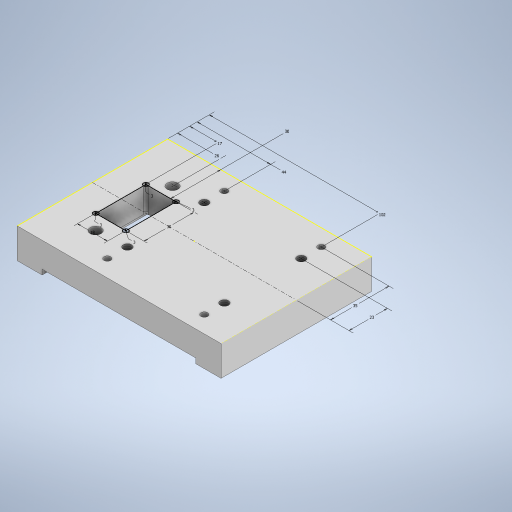
# Autodesk Inventor part: 05-15-2023 esercizi_iogna_serie
Saved by Autodesk Inventor 2023 (Build 270158000, 158)
## iProperties
Created: 2023-05-15
Part Number: 05-15-2023 esercizi_iogna_serie
Material: Generico
Document SubType Name: Modeling
Designer: Admin
Density: 1 g/cm^3
Appearance: Default
Author: Admin
Autodesk Inventor part; units mm, degrees
ref_plane "YZ Plane" through (0, 0, 0) normal (1, 0, 0) x (0, 1, 0)
ref_plane "XZ Plane" through (0, 0, 0) normal (0, 1, 0) x (-1, 0, 0)
ref_plane "XY Plane" through (0, 0, 0) normal (0, 0, 1) x (1, 0, 0)
sketch "Schizzo3" plane through (0, 0, 0) normal (0, 0, 1) x (1, 0, 0)
  line L0 (-46, 0) -> (-46, 3)
  line L1 (-46, 3) -> (46, 3)
  line L2 (46, 3) -> (46, 0)
  line L3 (46, 0) -> (61, 0)
  line L4 (61, 0) -> (61, 18)
  line L5 (61, 18) -> (-61, 18)
  line L6 (-61, 18) -> (-61, 0)
  line L7 (-61, 0) -> (-46, 0)
  line L8 (0, 0) -> (0, 18)
  point P0 (0, 3)
  dimension "d10" = 122
  dimension "d11" = 92
  dimension "d12" = 18
  dimension "d13" = 3
  constraints: 18 end point, 8 perpendicular, 2 midpoint, 2 point on line, 1 horizontal alignment, 1 vertical
  measures "d10" distance of L4.end L5.end
  measures "d11" distance of L0.end L1.end
  measures "d12" distance of L3.end L4.end
  measures "d13" distance of L1.end L2.end
extrude "Estrusione1" add sketch "Schizzo3" along normal mid plane 90
sketch "Schizzo4" plane through (-61, 18, 45) normal (0, 1, 0) x (1, 0, 0)
  line L0 (0, 90) -> (0, 0) projected
  line L1 (0, 90) -> (122, 90) projected
  line L2 (17, 60) -> (35, 60)
  line L3 (35, 60) -> (35, 30)
  line L4 (35, 30) -> (17, 30)
  line L5 (17, 30) -> (17, 60)
  line L6 (0, 45) -> (122, 45) construction
  line L7 (122, 90) -> (122, 0) construction
  circle A0 centre (17, 60) radius 1.5
  circle A1 centre (35, 60) radius 1.5
  circle A2 centre (35, 30) radius 1.5
  circle A3 centre (17, 30) radius 1.5
  point P0 (61, 45)
  point P1 (26, 68)
  point P2 (44, 80)
  point P3 (44, 68)
  point P4 (102, 80)
  point P5 (102, 68)
  point P6 (18.5, 30)
  point P7 (33.5, 30)
  point P8 (35, 31.5)
  point P9 (35, 58.5)
  point P10 (33.5, 60)
  point P11 (18.5, 60)
  point P12 (17, 58.5)
  point P13 (17, 31.5)
  dimension "d17" = 17
  dimension "d18" = 30
  dimension "d19" = 18
  dimension "d20" = 30
  dimension "d22" = 35
  dimension "d23" = 102
  dimension "d24" = 23
  dimension "d25" = 44
  dimension "d26" = 26
  dimension "d27" = 3
  dimension "d28" = 3
  dimension "d29" = 3
  dimension "d30" = 3
  constraints: 10 end point, 4 centre point, 4 coincident, 3 horizontal alignment, 2 midpoint, 2 parallel, 2 vertical alignment, 1 horizontal, 1 perpendicular
  measures "d17" distance from line of L2.start L0
  measures "d18" distance from line of L1 L2.start
  measures "d19" distance of L3.end L4.end
  measures "d20" distance of L2.end L3.end
  measures "d22" distance from line of point (102, 80) L6
  measures "d23" distance from line of point (102, 80) L0
  measures "d24" distance from line of point (102, 68) L6
  measures "d25" distance from line of L0 point (44, 80)
  measures "d26" distance from line of L0 point (26, 68)
  measures "d27" diameter of A0
  measures "d28" diameter of A1
  measures "d29" diameter of A2
  measures "d30" diameter of A3
extrude "Estrusione2" cut sketch "Schizzo4" against normal blind 90
hole "Foro1" at (41, 18, -23) at (-17, 18, -23) direction (0, -1, 0) diameter 4.917 end through all thread size "M6x1" class "6H" standard "ISO Metric profile"
hole "Foro2" at (41, 18, -35) at (-17, 18, -35) direction (0, -1, 0) diameter 4 end through all
pattern_linear "Serie rettangolare1" count 2 spacing 46 along (0, 0, 1) of "Foro1"
pattern_linear "Serie rettangolare2" count 2 spacing 70 along (0, 0, 1) of "Foro2"
sketch "Schizzo5" plane through (-46, 3, 45) normal (0, -1, 0) x (1, 0, 0)
  line L0 (-15, -90) -> (-15, 0) projected
  line L1 (92, -90) -> (0, -90) projected
  point P0 (46, -45)
  point P1 (11, -67)
  dimension "d54" = 26
  dimension "d55" = 23
  measures "d54" distance from line of L0 point (11, -67)
  measures "d55" distance from line of L1 point (11, -67)
hole "Foro3" at (-35, 3, -22) direction (0, 1, 0) diameter 6.5 end through all counterbore diameter 11 counterbore depth 6.5
pattern_linear "Serie rettangolare3" count 2 spacing 46 along (0, 0, 1) of "Foro3"
